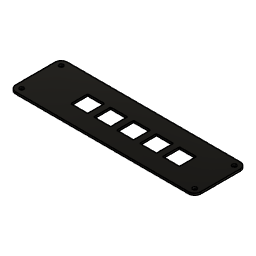
bottomcase (Autodesk Fusion 360 design; units mm, degrees)
Autodesk Fusion 360 part; units mm, degrees
sketch "plate-2025-06-26T05_56_28.958Z" plane through (0, 0, 0) normal (0, 0, 1) x (1, 0, 0)
  line L0 (22.075, -2.525) -> (35.075, -2.525)
  line L1 (22.075, -16.525) -> (35.075, -16.525)
  line L2 (21.575, -3.025) -> (21.575, -16.025)
  line L3 (35.575, -3.025) -> (35.575, -16.025)
  arc A0 (22.075, -2.525) -> (21.575, -3.025) centre (22.075, -3.025) ccw
  arc A1 (35.575, -3.025) -> (35.075, -2.525) centre (35.075, -3.025) ccw
  arc A2 (21.575, -16.025) -> (22.075, -16.525) centre (22.075, -16.025) ccw
  arc A3 (35.075, -16.525) -> (35.575, -16.025) centre (35.075, -16.025) ccw
  line L4 (41.125, -2.525) -> (54.125, -2.525)
  line L5 (41.125, -16.525) -> (54.125, -16.525)
  line L6 (40.625, -3.025) -> (40.625, -16.025)
  line L7 (54.625, -3.025) -> (54.625, -16.025)
  arc A4 (41.125, -2.525) -> (40.625, -3.025) centre (41.125, -3.025) ccw
  arc A5 (54.625, -3.025) -> (54.125, -2.525) centre (54.125, -3.025) ccw
  arc A6 (40.625, -16.025) -> (41.125, -16.525) centre (41.125, -16.025) ccw
  arc A7 (54.125, -16.525) -> (54.625, -16.025) centre (54.125, -16.025) ccw
  line L8 (60.175, -2.525) -> (73.175, -2.525)
  line L9 (60.175, -16.525) -> (73.175, -16.525)
  line L10 (59.675, -3.025) -> (59.675, -16.025)
  line L11 (73.675, -3.025) -> (73.675, -16.025)
  arc A8 (60.175, -2.525) -> (59.675, -3.025) centre (60.175, -3.025) ccw
  arc A9 (73.675, -3.025) -> (73.175, -2.525) centre (73.175, -3.025) ccw
  arc A10 (59.675, -16.025) -> (60.175, -16.525) centre (60.175, -16.025) ccw
  arc A11 (73.175, -16.525) -> (73.675, -16.025) centre (73.175, -16.025) ccw
  line L12 (138.92, -30.97) -> (-14.8, -30.97)
  line L13 (-14.8, -30.97) -> (-14.8, 11.89)
  line L14 (-14.8, 11.89) -> (138.92, 11.89)
  line L15 (138.92, 11.89) -> (138.92, -30.97)
  line L16 (128.92, 1.89) -> (-4.8, 1.89)
  line L17 (-4.8, 1.89) -> (-4.8, -20.97)
  line L18 (-4.8, -20.97) -> (128.92, -20.97)
  line L19 (128.92, -20.97) -> (128.92, 1.89)
  circle A12 centre (133.92, 6.89) radius 1.7
  circle A13 centre (133.92, -25.97) radius 1.7
  circle A14 centre (-9.8, -25.97) radius 1.7
  circle A15 centre (-9.8, 6.89) radius 1.7
  arc A16 (54.625, -3.025) -> (54.125, -2.525) centre (54.125, -3.025) ccw
  line L20 (21.575, -3.025) -> (21.575, -16.025)
  arc A17 (60.175, -2.525) -> (59.675, -3.025) centre (60.175, -3.025) ccw
  arc A18 (54.125, -16.525) -> (54.625, -16.025) centre (54.125, -16.025) ccw
  line L21 (40.625, -3.025) -> (40.625, -16.025)
  line L22 (35.575, -3.025) -> (35.575, -16.025)
  line L23 (59.675, -3.025) -> (59.675, -16.025)
  line L24 (22.075, -16.525) -> (35.075, -16.525)
  line L25 (41.125, -16.525) -> (54.125, -16.525)
  arc A19 (41.125, -2.525) -> (40.625, -3.025) centre (41.125, -3.025) ccw
  line L26 (60.175, -2.525) -> (73.175, -2.525)
  line L27 (54.625, -3.025) -> (54.625, -16.025)
  arc A20 (22.075, -2.525) -> (21.575, -3.025) centre (22.075, -3.025) ccw
  arc A21 (73.675, -3.025) -> (73.175, -2.525) centre (73.175, -3.025) ccw
  line L28 (73.675, -3.025) -> (73.675, -16.025)
  arc A22 (35.075, -16.525) -> (35.575, -16.025) centre (35.075, -16.025) ccw
  arc A23 (35.575, -3.025) -> (35.075, -2.525) centre (35.075, -3.025) ccw
  arc A24 (21.575, -16.025) -> (22.075, -16.525) centre (22.075, -16.025) ccw
  line L29 (60.175, -16.525) -> (73.175, -16.525)
  arc A25 (59.675, -16.025) -> (60.175, -16.525) centre (60.175, -16.025) ccw
  arc A26 (40.625, -16.025) -> (41.125, -16.525) centre (41.125, -16.025) ccw
  line L30 (41.125, -2.525) -> (54.125, -2.525)
  arc A27 (73.175, -16.525) -> (73.675, -16.025) centre (73.175, -16.025) ccw
  line L31 (22.075, -2.525) -> (35.075, -2.525)
  line L32 (79.225, -2.525) -> (92.225, -2.525)
  line L33 (98.275, -2.525) -> (111.275, -2.525)
  arc A28 (111.275, -16.525) -> (111.775, -16.025) centre (111.275, -16.025) ccw
  line L34 (111.775, -3.025) -> (111.775, -16.025)
  arc A29 (111.775, -3.025) -> (111.275, -2.525) centre (111.275, -3.025) ccw
  arc A30 (111.275, -16.525) -> (111.775, -16.025) centre (111.275, -16.025) ccw
  line L35 (79.225, -16.525) -> (92.225, -16.525)
  line L36 (98.275, -2.525) -> (111.275, -2.525)
  line L37 (98.275, -16.525) -> (111.275, -16.525)
  arc A31 (79.225, -2.525) -> (78.725, -3.025) centre (79.225, -3.025) ccw
  arc A32 (92.225, -16.525) -> (92.725, -16.025) centre (92.225, -16.025) ccw
  arc A33 (111.775, -3.025) -> (111.275, -2.525) centre (111.275, -3.025) ccw
  arc A34 (97.775, -16.025) -> (98.275, -16.525) centre (98.275, -16.025) ccw
  arc A35 (98.275, -2.525) -> (97.775, -3.025) centre (98.275, -3.025) ccw
  arc A36 (92.225, -16.525) -> (92.725, -16.025) centre (92.225, -16.025) ccw
  line L38 (111.775, -3.025) -> (111.775, -16.025)
  line L39 (97.775, -3.025) -> (97.775, -16.025)
  line L40 (98.275, -16.525) -> (111.275, -16.525)
  arc A37 (79.225, -2.525) -> (78.725, -3.025) centre (79.225, -3.025) ccw
  line L41 (92.725, -3.025) -> (92.725, -16.025)
  arc A38 (92.725, -3.025) -> (92.225, -2.525) centre (92.225, -3.025) ccw
  line L42 (78.725, -3.025) -> (78.725, -16.025)
  line L43 (97.775, -3.025) -> (97.775, -16.025)
  arc A39 (78.725, -16.025) -> (79.225, -16.525) centre (79.225, -16.025) ccw
  line L44 (92.725, -3.025) -> (92.725, -16.025)
  line L45 (79.225, -2.525) -> (92.225, -2.525)
  arc A40 (97.775, -16.025) -> (98.275, -16.525) centre (98.275, -16.025) ccw
  arc A41 (92.725, -3.025) -> (92.225, -2.525) centre (92.225, -3.025) ccw
  arc A42 (98.275, -2.525) -> (97.775, -3.025) centre (98.275, -3.025) ccw
  line L46 (78.725, -3.025) -> (78.725, -16.025)
  arc A43 (78.725, -16.025) -> (79.225, -16.525) centre (79.225, -16.025) ccw
  line L47 (79.225, -16.525) -> (92.225, -16.525)
  dimension "d1" = 153.72
  dimension "d2" = 42.86
  dimension "d9" = 10
  dimension "d11" = 5.05
  dimension "d12" = 5.05
  dimension "d13" = 3.4
  dimension "d14" = 3.4
  dimension "d15" = 3.4
  dimension "d16" = 3.4
  dimension "d17" = 5
  dimension "d18" = 5
  dimension "d19" = 5
  dimension "d20" = 5
  dimension "d21" = 5
  dimension "d22" = 5
  dimension "d23" = 5
  dimension "d24" = 5
  dimension "d29" = 10
  dimension "d30" = 10
  dimension "d31" = 10
  dimension "d32" = 26.375
  dimension "d33" = 5.05
  dimension "d34" = 5.05
  dimension "d35" = 5.05
  dimension "d36" = 5.05
  constraint horizontal L12
  constraint vertical L13
  constraint horizontal L14
  constraint vertical L15
  constraint horizontal L16
  constraint vertical L17
  constraint horizontal L18
  constraint vertical L19
  measures "d1" distance of L12.start L12.end
  measures "d2" distance of L12.start L14.end
  measures "d9" distance of L12 L18
  measures "d11" distance of L7 L10
  measures "d12" distance of L3 L6
  measures "d13" diameter of A12
  measures "d14" diameter of A13
  measures "d15" diameter of A14
  measures "d16" diameter of A15
  measures "d17" distance of L14 A15.centre
  measures "d18" distance of L13 A15.centre
  measures "d19" distance of L13 A14.centre
  measures "d20" distance of L12 A14.centre
  measures "d21" distance of L15 A13.centre
  measures "d22" distance of L12 A13.centre
  measures "d23" distance of L15 A12.centre
  measures "d24" distance of L14 A12.centre
  measures "d29" distance of L13 L17
  measures "d30" distance of L15 L19
  measures "d31" distance of L14 L16
  measures "d32" distance of L2 L17
  measures "d33" distance of L23 L27
  measures "d34" distance of L21 L22
  measures "d35" distance of L43 L44
  measures "d36" distance of L39 L41
extrude "Extrude1" add sketch "plate-2025-06-26T05_56_28.958Z" along normal blind 1.5 contours L12 L13 L14 L15 | L16 L17 L18 L19
fillet "Fillet1" radius 5 4 edges at (138.92, -30.97, 0.75) (138.92, 11.89, 0.75) (-14.8, -30.97, 0.75) (-14.8, 11.89, 0.75)
equation "d1 = 115.620 mm + 38.1 mm"
